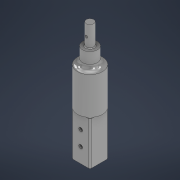
# Autodesk Inventor part: member_s2c
Saved by Autodesk Inventor 2021 (Build 250183000, 183)
## iProperties
Created: 2021-06-22
Part Number: member_s2c
Material: Generic High Carbon Steel
Document SubType Name: Modeling
Designer: Watchdog
Density: 7.5 g/cm^3
Appearance: Generic
Mass: 511.606 g
Surface Area: 198.285 cm^2
Volume: 68.2141 cm^3
Author: Watchdog
Autodesk Inventor part; units mm, degrees
ref_plane "YZ Plane" through (0, 0, 0) normal (1, 0, 0) x (0, 1, 0)
sketch "Sketch1" plane through (0, 0, 0) normal (0, 1, 0) x (-1, 0, 0)
  line L0 (12.5, -12.5) -> (-12.5, -12.5)
  line L1 (-12.5, -12.5) -> (-12.5, 12.5)
  line L2 (-12.5, 12.5) -> (12.5, 12.5)
  line L3 (12.5, 12.5) -> (12.5, -12.5)
  line L4 (10, 10) -> (-10, 10)
  line L5 (-10, 10) -> (-10, -10)
  line L6 (-10, -10) -> (10, -10)
  line L7 (10, -10) -> (10, 10)
  point P0 (0, 0)
  dimension "d0" = 25
  dimension "d1" = 25
  dimension "d2" = 12.5
  dimension "d3" = 12.5
  dimension "d4" = 2.5
  constraints: 16 end point, 4 parallel, 2 perpendicular, 1 horizontal, 3 other
  measures "d0" distance of L0.start L0.end
  measures "d1" distance of L0.end L1.end
  measures "d2" distance from line of point (0, 0) L0
  measures "d3" distance from line of L3 point (0, 0)
  measures "d4" distance between parallel lines of L2 L4
extrude "Extrusion1" add sketch "Sketch1" along normal blind 60
fillet "Fillet1" radius 2 4 edges at (-12.5, 30, 12.5) (12.5, 30, 12.5) (12.5, 30, -12.5) (-12.5, 30, -12.5)
sketch "Sketch2" plane through (0, 60, 0) normal (0, 1, 0) x (1, 0, 0)
  circle A0 centre (0, 0) radius 16.9706
  dimension "d8" = 33.9411
  constraints: 1 centre point, 1 coincident
  measures "d8" diameter of A0
extrude "Extrusion2" add sketch "Sketch2" along normal blind 50
sketch "Sketch3" plane through (0, 110, 0) normal (0, 1, 0) x (1, 0, 0)
  point P0 (0, 0)
sketch "Sketch4" plane through (0, 110, 0) normal (0, 1, 0) x (1, 0, 0)
  circle A0 centre (0, 0) radius 5
  dimension "d11" = 10
  constraints: 1 centre point, 1 coincident
  measures "d11" diameter of A0
extrude "Extrusion3" add sketch "Sketch4" along normal blind 50
ref_plane "Work Plane1" through (0, 110, 5) normal (0, 0, 1) x (1, 0, 0)
sketch "Sketch5" plane through (0, 110, 5) normal (0, 0, 1) x (1, 0, 0)
  line L0 (5, 50) -> (-5, 50) projected
  line L1 (-12.5, -50) -> (-12.5, -110) projected
  point P0 (0, -110)
  point P1 (0, 35)
  point P2 (0, 0)
  dimension "d19" = 12.5
  dimension "d28" = 15
  measures "d19" distance from line of point (0, 35) L1
  measures "d28" distance from line of L0 point (0, 35)
hole "Hole1" at (0, 145, 5) direction (0, 0, -1) diameter 3.242 end through all thread size "M4x0.7" class "6H" standard "ISO Metric profile"
ref_plane "Work Plane2" through (0, 132, 0) normal (0, 1, 0) x (1, 0, 0)
sketch "Sketch6" plane through (0, 132, 0) normal (0, 1, 0) x (1, 0, 0)
  circle A0 centre (0, 0) radius 5 projected
  circle A1 centre (0, 0) radius 10
  dimension "d30" = 5
  constraints: 1 centre point
  measures "d30" radial gap between concentric circles of A0 A1
extrude "Extrusion4" add sketch "Sketch6" against normal up to surface (22 mm away) contours A0 | A1
fillet "Fillet3" radius 1 1 edges at (-5, 132, 0)
fillet "Fillet4" radius 7 1 edges at (-10, 110, 0)
sketch "Sketch7" plane through (-10.5, 0, 12.5) normal (0, 0, 1) x (1, 0, 0)
  point P0 (10.5, 0)
  point P1 (10.5, 20)
  point P2 (10.5, 40)
  dimension "d35" = 0
  dimension "d36" = 0
  dimension "d37" = 20
  dimension "d38" = 20
  measures "d35" horizontal distance of point (10.5, 0) point (10.5, 20)
  measures "d36" horizontal distance of point (10.5, 0) point (10.5, 40)
  measures "d37" distance of point (10.5, 0) point (10.5, 20)
  measures "d38" distance of point (10.5, 20) point (10.5, 40)
hole "Hole2" at (0, 40, 12.5) at (0, 20, 12.5) direction (0, 0, -1) diameter 5 end through all
fillet "Fillet5" radius 2 8 edges at (-11.9142, 60, -11.9142) (-12.5, 60, 0) (-11.9142, 60, 11.9142) (0, 60, 12.5) (11.9142, 60, 11.9142) (12.5, 60, 0) (11.9142, 60, -11.9142) (0, 60, -12.5)
equation "\"d1\" = d0"
equation "\"d2\" = 0.5 * d1"
equation "\"d3\" = 0.5 * d0"
equation "\"d38\" = d37"
body "Solid1"
